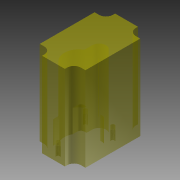
# Autodesk Inventor part: 13_1087_013
Saved by Autodesk Inventor 2014 SP1 (Build 180222100, 222)
## iProperties
Created: 2013-08-08
Part Number: 13_1087_013
Material: PPS-Kunststoff
Document SubType Name: Modeling
Designer: vogel
Density: 1.637 g/cm^3
Appearance: Klar - gelb
Author: vogel
Autodesk Inventor part; units mm, degrees
ref_plane "YZ Plane" through (0, 0, 0) normal (1, 0, 0) x (0, 1, 0)
ref_plane "XZ Plane" through (0, 0, 0) normal (0, 1, 0) x (-1, 0, 0)
ref_plane "XY Plane" through (0, 0, 0) normal (0, 0, 1) x (1, 0, 0)
sketch "Skizze1" plane through (0, 0, 0) normal (0, 0, 1) x (1, 0, 0)
  line L0 (-14, 0) -> (14, 0) projected
  line L1 (0, -15.4) -> (0, 15.4) projected
  line L2 (-10, 11) -> (10, 11)
  line L3 (10, 11) -> (10, -11)
  line L4 (10, -11) -> (-10, -11)
  line L5 (-10, -11) -> (-10, 11)
  point P0 (0, 0)
  dimension "d0" = 22
  dimension "d1" = 20
  constraints: 8 end point, 2 parallel, 1 horizontal, 1 perpendicular, 2 other
  measures "d0" distance of L4.end L2.start
  measures "d1" distance of L3.end L4.end
extrude "Extrusion1" add sketch "Skizze1" along normal blind 37
sketch "Skizze2" plane through (0, 0, 0) normal (0, 0, -1) x (-1, 0, 0)
  point P0 (0, 0)
hole "Bohrung1" at (0, 0, 0) direction (0, 0, 1) diameter 12.5 depth 32 tip angle 118
sketch "Skizze3" plane through (0, 0, 0) normal (0, 0, -1) x (-1, 0, 0)
  line L0 (14, 0) -> (-14, 0) projected
  line L1 (0, -15.4) -> (0, 15.4) projected
  line L2 (-5.5, 6.5) -> (5.5, 6.5)
  line L3 (5.5, 6.5) -> (5.5, -6.5)
  line L4 (5.5, -6.5) -> (-5.5, -6.5)
  line L5 (-5.5, -6.5) -> (-5.5, 6.5)
  dimension "d11" = 13
  dimension "d12" = 11
  constraints: 8 end point, 2 parallel, 1 horizontal, 1 perpendicular, 2 other
  measures "d11" distance of L4.end L2.start
  measures "d12" distance of L3.end L4.end
extrude "Extrusion2" cut sketch "Skizze3" against normal blind 10
fillet "Rundung1" radius 1.5 4 edges at (-5.5, -6.5, 5) (-5.5, 6.5, 5) (5.5, 6.5, 5) (5.5, -6.5, 5)
sketch "Skizze4" plane through (0, 0, 37) normal (0, 0, 1) x (1, 0, 0)
  line L0 (-10, 11) -> (-10, -11) projected
  line L1 (-10, -11) -> (10, -11) projected
  line L2 (-4, -6.5) -> (4, -6.5) projected
  arc A0 (4, -6.5) -> (5.5, -5) centre (4, -5) ccw projected
  line L3 (5.5, -5) -> (5.5, -2.9686) projected
  arc A1 (-5.5, -5) -> (-4, -6.5) centre (-4, -5) ccw projected
  line L4 (-5.5, -2.9686) -> (-5.5, -5) projected
  line L5 (-10, -7) -> (-5, -7)
  line L6 (-5, -7) -> (-5, -11)
  line L7 (-5, -11) -> (-10, -11)
  line L8 (-10, -11) -> (-10, -7)
  line L9 (10, -11) -> (5, -11)
  line L10 (5, -11) -> (5, -7)
  line L11 (5, -7) -> (10, -7)
  line L12 (10, -7) -> (10, -11)
  point P0 (0, 0)
  dimension "d16" = 5
  dimension "d17" = 4
  dimension "d18" = 5
  constraints: 16 end point, 4 parallel, 2 horizontal, 2 perpendicular, 2 point on line, 1 collinear
  measures "d16" distance between parallel lines of L6 L8
  measures "d17" distance between parallel lines of L5 L1
  measures "d18" distance between parallel lines of L12 L10
extrude "Extrusion3" cut sketch "Skizze4" against normal through all
fillet "Rundung2" radius 3 2 edges at (-5, -7, 18.5) (5, -7, 18.5)
sketch "Skizze5" plane through (-10, 11, 0) normal (0, 1, 0) x (1, 0, 0)
  line L0 (0, 0) -> (20, 0) projected
  line L1 (0, 0) -> (20, 0)
  line L2 (20, 0) -> (20, -10)
  line L3 (20, -10) -> (0, -10)
  line L4 (0, -10) -> (0, 0)
  line L5 (-4, 0) -> (24, 0) projected
  line L6 (10, 7.4) -> (10, -44.4) projected
  point P0 (10, 0)
  dimension "d22" = 20
  dimension "d23" = 10
  constraints: 8 end point, 2 parallel, 1 horizontal, 1 perpendicular, 1 point on line, 1 other
  measures "d22" distance of L2.end L3.end
  measures "d23" distance between parallel lines of L0 L3
extrude "Extrusion4" add sketch "Skizze5" along normal blind 10
sketch "Skizze7" plane through (0, 0, 0) normal (0, 0, -1) x (-1, 0, 0)
  circle A0 centre (-6, 9) radius 1.2 projected
  circle A1 centre (6, 9) radius 1.2 projected
  circle A2 centre (0, -9) radius 1.2 projected
  constraints: 3 coincident
hole "Bohrung3" at (6, 9, 0) at (-6, 9, 0) at (0, -9, 0) direction (0, 0, 1) diameter 1.567 depth 6 tip angle 118 thread size "M2x0.4" class "6H" standard "ISO Metric profile"
sketch "Skizze8" plane through (-10, 11, 37) normal (0, 1, 0) x (1, 0, 0)
  line L0 (20, 27) -> (0, 27) projected
  line L1 (0, 27) -> (0, 0) projected
  line L2 (20, 0) -> (0, 0) projected
  line L3 (20, 27) -> (20, 0) projected
  point P0 (10, 37)
extrude "Extrusion5" add sketch "Skizze8" along normal blind 6
sketch "Skizze9" plane through (-10, 21, 10) normal (0, 0, 1) x (1, 0, 0)
  line L0 (20, -4) -> (20, 0) projected
  line L1 (0, 0) -> (20, 0) projected
  circle A0 centre (4, -12) radius 1.2 projected
  circle A1 centre (16, -12) radius 1.2 projected
  circle A2 centre (10, -30) radius 1.2 projected
  circle A3 centre (18, -1) radius 2.25 projected
  circle A4 centre (18, -31) radius 2.25 projected
  circle A5 centre (2, -31) radius 2.25 projected
  circle A6 centre (2, -1) radius 2.25 projected
  circle A7 centre (13, -17) radius 1.75 projected
  circle A8 centre (7, -25) radius 1.75 projected
  circle A9 centre (10, -25.5) radius 0.9 projected
  circle A10 centre (10, -16.5) radius 0.9 projected
  circle A11 centre (10, -21) radius 3 projected
  line L2 (23, 2) -> (-3, 2) projected
  line L3 (-3, 2) -> (-3, -34) projected
  line L4 (-3, -34) -> (23, -34) projected
  line L5 (23, 2) -> (23, -34) projected
  line L6 (15, 0) -> (20, 0)
  line L7 (20, 0) -> (20, -4)
  line L8 (20, -4) -> (15, -4)
  line L9 (15, -4) -> (15, 0)
  line L10 (0, 0) -> (5, 0)
  line L11 (5, 0) -> (5, -4)
  line L12 (5, -4) -> (0, -4)
  line L13 (0, -4) -> (0, 0)
  line L14 (10, 0) -> (10, -17.7524)
  circle A12 centre (10, -12) radius 3 projected
  point P0 (10, -21)
  dimension "d44" = 3
  dimension "d45" = 3
  constraints: 18 end point, 5 parallel, 2 collinear, 2 horizontal, 2 perpendicular, 1 midpoint, 1 point on line, 1 other
  measures "d44" distance from line of L9 A3.centre
  measures "d45" distance from line of L8 A3.centre
extrude "Extrusion6" cut sketch "Skizze9" against normal through all contours L8 L9 L1 A3 L0 | L11 L12 L13 A6 L1 | A3 L1 L0 | A6 L13 L1 picked at (17.2844, -1.2206) picked at (2.725, -1.1961)
fillet "Rundung3" radius 3 2 edges at (5, 17, 5) (-5, 17, 5)
sketch "Skizze10" plane through (0, 0, 0) normal (0, 0, -1) x (-1, 0, 0)
  line L0 (-5.5, -5) -> (-5.5, -2.9686) projected
  arc A0 (2, 11.2361) -> (-2, 11.2361) centre (0, 9) ccw projected
  arc A1 (-2, 11.2361) -> (2, 11.2361) centre (0, 9) ccw projected
  arc A2 (3, 9) -> (-3, 9) centre (0, 9) ccw
  line L1 (-3, 9) -> (-3, 4)
  line L2 (-3, 4) -> (3, 4)
  line L3 (3, 9) -> (3, 4)
  arc A3 (5.5, 2.9686) -> (-5.5, 2.9686) centre (0, 0) ccw projected
  dimension "d49" = 3
  dimension "d50" = 5
  constraints: 6 end point, 2 coincident, 2 perpendicular, 2 point on circle, 2 tangent, 1 centre point, 1 parallel
  measures "d49" radius of A2
  measures "d50" distance from line of L2 point (0, 9)
extrude "Extrusion7" cut sketch "Skizze10" against normal blind 32
sketch "Skizze11" plane through (-5, 21, 10) normal (0, 0, 1) x (1, 0, 0)
  line L0 (0, 0) -> (0, -1) projected
  arc A0 (-3, -4) -> (0, -1) centre (-3, -1) ccw projected
  line L1 (-3, -4) -> (13, -4) projected
  arc A1 (10, -1) -> (13, -4) centre (13, -1) ccw projected
  line L2 (10, -1) -> (10, 0) projected
  line L3 (0, 0) -> (10, 0) projected
  point P0 (5, -21)
extrude "Extrusion8" add sketch "Skizze11" along normal up to surface (27 mm away)
